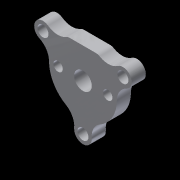
# Autodesk Inventor part: Pnuematic Plate
Saved by Autodesk Inventor 2014 SP1 (Build 180222100, 222)
## iProperties
Created: 2014-01-20
Part Number: Pnuematic Plate
Material: Aluminum 6061
Document SubType Name: Modeling
Designer: Rauhul Varma
Mass: 13.9422 g
Surface Area: 31.2131 cm^2
Volume: 5.14472 cm^3
Density: 2.71 g/cm^3
Appearance: Aluminum - Flat
Author: Rauhul Varma
Autodesk Inventor part; units mm, degrees
ref_plane "YZ Plane" through (0, 0, 0) normal (1, 0, 0) x (0, 1, 0)
ref_plane "XZ Plane" through (0, 0, 0) normal (0, 1, 0) x (-1, 0, 0)
ref_plane "XY Plane" through (0, 0, 0) normal (0, 0, 1) x (1, 0, 0)
sketch "Sketch1" plane through (0, 0, 0) normal (0, 0, 1) x (1, 0, 0)
  circle A0 centre (0, 0) radius 20.7359 construction
  line L0 (0, 0) -> (-17.9578, 10.368) construction
  arc A1 (-19.6042, 6.7568) -> (-15.6537, 13.5993) centre (-17.9578, 10.368) ccw construction
  arc A2 (-7.603, 13.208) -> (-15.24, -0.0196) centre (0, 0) ccw construction
  arc A3 (-15.24, -0.0196) -> (-19.6042, 6.7568) centre (-22.698, -0.0292) ccw
  arc A4 (-15.6537, 13.5993) -> (-7.603, 13.208) centre (-11.3237, 19.6716) ccw
  line L1 (0, 0) -> (-20.7359, 0) construction
  arc A5 (-15.6537, 13.5993) -> (-19.6042, 6.7568) centre (-17.9578, 10.368) ccw
  arc A6 (-15.24, -0.0196) -> (-7.637, -13.1884) centre (0, 0) ccw
  arc A7 (7.637, -13.1884) -> (3.9505, -20.3561) centre (11.3743, -19.6424) ccw
  arc A8 (-3.9505, -20.3561) -> (-7.637, -13.1884) centre (-11.3743, -19.6424) ccw
  arc A9 (-3.9505, -20.3561) -> (3.9505, -20.3561) centre (0, -20.7359) ccw
  arc A10 (7.603, 13.208) -> (15.6537, 13.5993) centre (11.3237, 19.6716) ccw
  arc A11 (19.6042, 6.7568) -> (15.24, -0.0196) centre (22.698, -0.0292) ccw
  arc A12 (19.6042, 6.7568) -> (15.6537, 13.5993) centre (17.9578, 10.368) ccw
  arc A13 (7.603, 13.208) -> (6.643, 13.716) centre (0, 0) ccw
  arc A14 (7.637, -13.1884) -> (15.24, -0.0196) centre (0, 0) ccw
  arc A15 (-7.637, -13.1884) -> (7.637, -13.1884) centre (0, 0) ccw construction
  arc A16 (15.24, -0.0196) -> (7.603, 13.208) centre (0, 0) ccw construction
  circle A17 centre (0, 0) radius 3.9688
  circle A18 centre (0, 0) radius 11.176 construction
  line L2 (0, -20.7359) -> (0, 0) construction
  line L3 (0, 0) -> (11.176, 0) construction
  line L4 (-6.643, 13.716) -> (6.643, 13.716)
  arc A19 (-6.643, 13.716) -> (-7.603, 13.208) centre (0, 0) ccw
  arc A20 (6.643, 13.716) -> (-6.643, 13.716) centre (0, 0) ccw construction
  point P0 (-11.176, 0)
  dimension "d0" = 41.4719
  dimension "d3" = 7.9375
  dimension "d5" = 30
  dimension "d9" = 360
  dimension "d20" = 7.9375
  dimension "d21" = 22.352
  dimension "d22" = 15.24
  dimension "d23" = 13.716
  constraints: 43 point on circle, 21 centre point, 10 end point, 7 coincident, 4 tangent, 1 horizontal, 1 parallel, 1 perpendicular, 1 point on line, 31 other
  measures "d0" diameter of A0
  measures "d3" diameter of A1
  measures "d5" angle of L0 L1
  measures "d20" diameter of A17
  measures "d21" diameter of A18
  measures "d22" radius of A6
  measures "d23" distance from line of point (0, 0) L4
extrude "Extrusion1" add sketch "Sketch1" along normal blind 6.35
hole "Hole1" at (-17.9578, 10.368, 0) at (17.9578, 10.368, 0) at (0, -20.7359, 0) direction (0, 0, 1) diameter 4.9784 end through all clearance for "Socket Head Cap Screw" size "#10" standard "Ansi Unified Screw Threads"
hole "Hole2" at (-11.176, 0, 0) at (11.176, 0, 0) direction (0, 0, 1) diameter 4.2164 end through all
fillet "Fillet1" radius 3.175 2 edges at (-6.643, 13.716, 3.175) (6.643, 13.716, 3.175)
body "Solid1"
